Autodesk Fusion 360 part; units mm, degrees
note: some values were not read from the file. Set by a fixed rule: which sketch regions a step uses.
(part 3 of 3)
  spline S151 degree 3 poles (-49.2389, -12.8758) (-49.8818, -12.8354) (-50.64, -12.7486) (-51.5069, -12.5872) knots 0 0 0 0 1 1 1 1
  arc A152 (-51.6774, -11.868) -> (-51.5069, -12.5872) centre (0, 0) ccw
  spline S152 degree 3 poles (-51.6774, -11.868) (-50.9751, -11.3346) (-50.3365, -10.9168) (-49.7802, -10.5921) knots 0 0 0 0 1 1 1 1
  spline S153 degree 3 poles (-49.7802, -10.5921) (-49.639, -10.5097) (-49.5032, -10.4334) (-49.3731, -10.3628) knots 0 0 0 0 1 1 1 1
  arc A153 (-49.3731, -10.3628) -> (-49.172, -9.9321) centre (-49.564, -10.0113) ccw
  arc A154 (-49.276, -9.4025) -> (-49.172, -9.9321) centre (0, 0) ccw
  arc A155 (-49.276, -9.4025) -> (-49.6251, -9.0799) centre (-49.6689, -9.4775) ccw
  spline S154 degree 3 poles (-49.6251, -9.0799) (-49.7722, -9.0637) (-49.9268, -9.0443) (-50.0886, -9.0215) knots 0 0 0 0 1 1 1 1
  spline S155 degree 3 poles (-50.0886, -9.0215) (-50.7265, -8.9313) (-51.4757, -8.786) (-52.3275, -8.5579) knots 0 0 0 0 1 1 1 1
  arc A156 (-52.4417, -7.8277) -> (-52.3275, -8.5579) centre (0, 0) ccw
  spline S156 degree 3 poles (-52.4417, -7.8277) (-51.7002, -7.3504) (-51.0311, -6.9833) (-50.4513, -6.7027) knots 0 0 0 0 1 1 1 1
  spline S157 degree 3 poles (-50.4513, -6.7027) (-50.3042, -6.6315) (-50.1629, -6.5659) (-50.0277, -6.5056) knots 0 0 0 0 1 1 1 1
  arc A157 (-50.0277, -6.5056) -> (-49.7938, -6.0917) centre (-50.1908, -6.1403) ccw
  arc A158 (-49.8564, -5.5557) -> (-49.7938, -6.0917) centre (0, 0) ccw
  arc A159 (-49.8564, -5.5557) -> (-50.1795, -5.207) centre (-50.254, -5.6) ccw
  spline S158 degree 3 poles (-50.1795, -5.207) (-50.3249, -5.1794) (-50.4775, -5.1482) (-50.6371, -5.1128) knots 0 0 0 0 1 1 1 1
  spline S159 degree 3 poles (-50.6371, -5.1128) (-51.266, -4.9735) (-52.0017, -4.7706) (-52.8333, -4.4772) knots 0 0 0 0 1 1 1 1
  arc A160 (-52.8906, -3.7403) -> (-52.8333, -4.4772) centre (0, 0) ccw
  spline S160 degree 3 poles (-52.8906, -3.7403) (-52.1143, -3.3219) (-51.4188, -3.0078) (-50.819, -2.773) knots 0 0 0 0 1 1 1 1
  spline S161 degree 3 poles (-50.819, -2.773) (-50.6668, -2.7134) (-50.5208, -2.6589) (-50.3814, -2.6092) knots 0 0 0 0 1 1 1 1
  arc A161 (-50.3814, -2.6092) -> (-50.1161, -2.2148) centre (-50.5157, -2.2324) ccw
  arc A162 (-50.137, -1.6755) -> (-50.1161, -2.2148) centre (0, 0) ccw
  arc A163 (-50.137, -1.6755) -> (-50.4321, -1.3028) centre (-50.5368, -1.6888) ccw
  spline S162 degree 3 poles (-50.4321, -1.3028) (-50.5749, -1.2641) (-50.7247, -1.2211) (-50.881, -1.1735) knots 0 0 0 0 1 1 1 1
  spline S163 degree 3 poles (-50.881, -1.1735) (-51.4973, -0.9858) (-52.215, -0.7265) (-53.0214, -0.3696) knots 0 0 0 0 1 1 1 1
  arc A164 (-53.0214, 0.3696) -> (-53.0214, -0.3696) centre (0, 0) ccw
  spline S164 degree 3 poles (-53.0214, 0.3696) (-52.215, 0.7265) (-51.4973, 0.9858) (-50.881, 1.1735) knots 0 0 0 0 1 1 1 1
  spline S165 degree 3 poles (-50.881, 1.1735) (-50.7247, 1.2211) (-50.5749, 1.2641) (-50.4321, 1.3028) knots 0 0 0 0 1 1 1 1
  arc A165 (-50.4321, 1.3028) -> (-50.137, 1.6755) centre (-50.5368, 1.6888) ccw
  arc A166 (-50.1161, 2.2148) -> (-50.137, 1.6755) centre (0, 0) ccw
  arc A167 (-50.1161, 2.2148) -> (-50.3814, 2.6092) centre (-50.5157, 2.2324) ccw
  spline S166 degree 3 poles (-50.3814, 2.6092) (-50.5208, 2.6589) (-50.6668, 2.7134) (-50.819, 2.773) knots 0 0 0 0 1 1 1 1
  spline S167 degree 3 poles (-50.819, 2.773) (-51.4188, 3.0078) (-52.1143, 3.3219) (-52.8906, 3.7403) knots 0 0 0 0 1 1 1 1
  arc A168 (-52.8333, 4.4772) -> (-52.8906, 3.7403) centre (0, 0) ccw
  spline S168 degree 3 poles (-52.8333, 4.4772) (-52.0017, 4.7706) (-51.266, 4.9735) (-50.6371, 5.1128) knots 0 0 0 0 1 1 1 1
  spline S169 degree 3 poles (-50.6371, 5.1128) (-50.4775, 5.1482) (-50.3249, 5.1794) (-50.1795, 5.207) knots 0 0 0 0 1 1 1 1
  arc A169 (-50.1795, 5.207) -> (-49.8564, 5.5557) centre (-50.254, 5.6) ccw
  arc A170 (-49.7938, 6.0917) -> (-49.8564, 5.5557) centre (0, 0) ccw
  arc A171 (-49.7938, 6.0917) -> (-50.0277, 6.5056) centre (-50.1908, 6.1403) ccw
  spline S170 degree 3 poles (-50.0277, 6.5056) (-50.1629, 6.5659) (-50.3042, 6.6315) (-50.4513, 6.7027) knots 0 0 0 0 1 1 1 1
  spline S171 degree 3 poles (-50.4513, 6.7027) (-51.0311, 6.9833) (-51.7002, 7.3504) (-52.4417, 7.8277) knots 0 0 0 0 1 1 1 1
  arc A172 (-52.3275, 8.5579) -> (-52.4417, 7.8277) centre (0, 0) ccw
  spline S172 degree 3 poles (-52.3275, 8.5579) (-51.4757, 8.786) (-50.7265, 8.9313) (-50.0886, 9.0215) knots 0 0 0 0 1 1 1 1
  spline S173 degree 3 poles (-50.0886, 9.0215) (-49.9268, 9.0443) (-49.7722, 9.0637) (-49.6251, 9.0799) knots 0 0 0 0 1 1 1 1
  arc A173 (-49.6251, 9.0799) -> (-49.276, 9.4025) centre (-49.6689, 9.4775) ccw
  arc A174 (-49.172, 9.9321) -> (-49.276, 9.4025) centre (0, 0) ccw
  arc A175 (-49.172, 9.9321) -> (-49.3731, 10.3628) centre (-49.564, 10.0113) ccw
  spline S174 degree 3 poles (-49.3731, 10.3628) (-49.5032, 10.4334) (-49.639, 10.5097) (-49.7802, 10.5921) knots 0 0 0 0 1 1 1 1
  spline S175 degree 3 poles (-49.7802, 10.5921) (-50.3365, 10.9168) (-50.9751, 11.3346) (-51.6774, 11.868) knots 0 0 0 0 1 1 1 1
  arc A176 (-51.5069, 12.5872) -> (-51.6774, 11.868) centre (0, 0) ccw
  spline S176 degree 3 poles (-51.5069, 12.5872) (-50.64, 12.7486) (-49.8818, 12.8354) (-49.2389, 12.8758) knots 0 0 0 0 1 1 1 1
  spline S177 degree 3 poles (-49.2389, 12.8758) (-49.0758, 12.8861) (-48.9202, 12.8934) (-48.7722, 12.8981) knots 0 0 0 0 1 1 1 1
  arc A177 (-48.7722, 12.8981) -> (-48.3992, 13.1927) centre (-48.7851, 13.2979) ccw
  arc A178 (-48.2544, 13.7127) -> (-48.3992, 13.1927) centre (0, 0) ccw
  arc A179 (-48.2544, 13.7127) -> (-48.4216, 14.1576) centre (-48.6392, 13.822) ccw
  spline S178 degree 3 poles (-48.4216, 14.1576) (-48.5458, 14.2382) (-48.6753, 14.3248) (-48.8097, 14.4179) knots 0 0 0 0 1 1 1 1
  spline S179 degree 3 poles (-48.8097, 14.4179) (-49.3392, 14.7847) (-49.9435, 15.2507) (-50.6023, 15.8369) knots 0 0 0 0 1 1 1 1
  arc A180 (-50.3766, 16.5407) -> (-50.6023, 15.8369) centre (0, 0) ccw
  spline S180 degree 3 poles (-50.3766, 16.5407) (-49.4998, 16.6345) (-48.7372, 16.6622) (-48.0931, 16.6527) knots 0 0 0 0 1 1 1 1
  spline S181 degree 3 poles (-48.0931, 16.6527) (-47.9296, 16.6503) (-47.7739, 16.6455) (-47.6261, 16.6388) knots 0 0 0 0 1 1 1 1
  arc A181 (-47.6261, 16.6388) -> (-47.2313, 16.9036) centre (-47.6079, 17.0384) ccw
  arc A182 (-47.0467, 17.4108) -> (-47.2313, 16.9036) centre (0, 0) ccw
  arc A183 (-47.0467, 17.4108) -> (-47.1789, 17.8674) centre (-47.4218, 17.5496) ccw
  spline S182 degree 3 poles (-47.1789, 17.8674) (-47.2965, 17.9573) (-47.4189, 18.0537) (-47.5456, 18.1569) knots 0 0 0 0 1 1 1 1
  spline S183 degree 3 poles (-47.5456, 18.1569) (-48.0451, 18.5637) (-48.6115, 19.0751) (-49.2229, 19.7105) knots 0 0 0 0 1 1 1 1
  arc A184 (-48.9434, 20.3948) -> (-49.2229, 19.7105) centre (0, 0) ccw
  spline S184 degree 3 poles (-48.9434, 20.3948) (-48.0619, 20.4203) (-47.2994, 20.3889) (-46.658, 20.3295) knots 0 0 0 0 1 1 1 1
  spline S185 degree 3 poles (-46.658, 20.3295) (-46.4952, 20.3145) (-46.3404, 20.2976) (-46.1935, 20.2794) knots 0 0 0 0 1 1 1 1
  arc A185 (-46.1935, 20.2794) -> (-45.7794, 20.5129) centre (-46.1444, 20.6764) ccw
  arc A186 (-45.556, 21.0042) -> (-45.7794, 20.5129) centre (0, 0) ccw
  arc A187 (-45.556, 21.0042) -> (-45.6525, 21.4697) centre (-45.9193, 21.1717) ccw
  spline S186 degree 3 poles (-45.6525, 21.4697) (-45.7627, 21.5684) (-45.8773, 21.674) (-45.9956, 21.7867) knots 0 0 0 0 1 1 1 1
  spline S187 degree 3 poles (-45.9956, 21.7867) (-46.4621, 22.231) (-46.9871, 22.7848) (-47.5475, 23.4657) knots 0 0 0 0 1 1 1 1
  arc A188 (-47.2158, 24.1262) -> (-47.5475, 23.4657) centre (0, 0) ccw
  spline S188 degree 3 poles (-47.2158, 24.1262) (-46.335, 24.0833) (-45.5772, 23.9929) (-44.9423, 23.884) knots 0 0 0 0 1 1 1 1
  spline S189 degree 3 poles (-44.9423, 23.884) (-44.7812, 23.8564) (-44.6281, 23.8276) (-44.4831, 23.7981) knots 0 0 0 0 1 1 1 1
  arc A189 (-44.4831, 23.7981) -> (-44.0521, 23.9987) centre (-44.4034, 24.1901) ccw
  arc A190 (-43.7914, 24.4713) -> (-44.0521, 23.9987) centre (0, 0) ccw
  arc A191 (-43.7914, 24.4713) -> (-43.8514, 24.9428) centre (-44.1406, 24.6664) ccw
  spline S190 degree 3 poles (-43.8514, 24.9428) (-43.9537, 25.0498) (-44.0597, 25.164) (-44.169, 25.2855) knots 0 0 0 0 1 1 1 1
  spline S191 degree 3 poles (-44.169, 25.2855) (-44.5997, 25.7646) (-45.0802, 26.3574) (-45.5861, 27.0797) knots 0 0 0 0 1 1 1 1
  arc A192 (-45.2042, 27.7125) -> (-45.5861, 27.0797) centre (0, 0) ccw
  spline S192 degree 3 poles (-45.2042, 27.7125) (-44.3294, 27.6015) (-43.5809, 27.4527) (-42.9563, 27.2949) knots 0 0 0 0 1 1 1 1
  spline S193 degree 3 poles (-42.9563, 27.2949) (-42.7979, 27.2549) (-42.6475, 27.2143) (-42.5051, 27.1736) knots 0 0 0 0 1 1 1 1
  arc A193 (-42.5051, 27.1736) -> (-42.0599, 27.3403) centre (-42.3953, 27.5583) ccw
  arc A194 (-41.7634, 27.7912) -> (-42.0599, 27.3403) centre (0, 0) ccw
  arc A195 (-41.7634, 27.7912) -> (-41.7867, 28.266) centre (-42.0964, 28.0128) ccw
  spline S194 degree 3 poles (-41.7867, 28.266) (-41.8804, 28.3806) (-41.9772, 28.5026) (-42.0767, 28.6322) knots 0 0 0 0 1 1 1 1
  spline S195 degree 3 poles (-42.0767, 28.6322) (-42.469, 29.1432) (-42.9021, 29.7715) (-43.3505, 30.5308) knots 0 0 0 0 1 1 1 1
  arc A196 (-42.9207, 31.1322) -> (-43.3505, 30.5308) centre (0, 0) ccw
  spline S196 degree 3 poles (-42.9207, 31.1322) (-42.0572, 30.9537) (-41.3225, 30.7473) (-40.712, 30.5416) knots 0 0 0 0 1 1 1 1
  spline S197 degree 3 poles (-40.712, 30.5416) (-40.5571, 30.4894) (-40.4103, 30.4373) (-40.2716, 30.3858) knots 0 0 0 0 1 1 1 1
  arc A197 (-40.2716, 30.3858) -> (-39.8148, 30.5174) centre (-40.1323, 30.7607) ccw
  arc A198 (-39.4842, 30.944) -> (-39.8148, 30.5174) centre (0, 0) ccw
  arc A199 (-39.4842, 30.944) -> (-39.4706, 31.4191) centre (-39.799, 31.1907) ccw
  spline S198 degree 3 poles (-39.4706, 31.4191) (-39.5552, 31.5406) (-39.6423, 31.6698) (-39.7314, 31.8068) knots 0 0 0 0 1 1 1 1
  spline S199 degree 3 poles (-39.7314, 31.8068) (-40.0829, 32.3466) (-40.466, 33.0066) (-40.8543, 33.7984) knots 0 0 0 0 1 1 1 1
  arc A200 (-40.3792, 34.3646) -> (-40.8543, 33.7984) centre (0, 0) ccw
  spline S200 degree 3 poles (-40.3792, 34.3646) (-39.532, 34.1197) (-38.8155, 33.857) (-38.2228, 33.6046) knots 0 0 0 0 1 1 1 1
  spline S201 degree 3 poles (-38.2228, 33.6046) (-38.0725, 33.5406) (-37.9301, 33.4773) (-37.7958, 33.4151) knots 0 0 0 0 1 1 1 1
  arc A201 (-37.7958, 33.4151) -> (-37.3302, 33.511) centre (-37.6279, 33.7782) ccw
  arc A202 (-36.9675, 33.9106) -> (-37.3302, 33.511) centre (0, 0) ccw
  arc A203 (-36.9675, 33.9106) -> (-36.9172, 34.3833) centre (-37.2623, 34.181) ccw
  spline S202 degree 3 poles (-36.9172, 34.3833) (-36.9921, 34.511) (-37.0689, 34.6465) (-37.1472, 34.79) knots 0 0 0 0 1 1 1 1
  spline S203 degree 3 poles (-37.1472, 34.79) (-37.4558, 35.3555) (-37.7866, 36.0432) (-38.1123, 36.8626) knots 0 0 0 0 1 1 1 1
  arc A204 (-37.5947, 37.3903) -> (-38.1123, 36.8626) centre (0, 0) ccw
  spline S204 degree 3 poles (-37.5947, 37.3903) (-36.7691, 37.0806) (-36.0751, 36.7631) (-35.5038, 36.4656) knots 0 0 0 0 1 1 1 1
  spline S205 degree 3 poles (-35.5038, 36.4656) (-35.3588, 36.3901) (-35.2218, 36.3159) (-35.0927, 36.2435) knots 0 0 0 0 1 1 1 1
  arc A205 (-35.0927, 36.2435) -> (-34.6211, 36.303) centre (-34.8972, 36.5925) ccw
  arc A206 (-34.2285, 36.6734) -> (-34.6211, 36.303) centre (0, 0) ccw
  arc A207 (-34.2285, 36.6734) -> (-34.1418, 37.1407) centre (-34.5015, 36.9658) ccw
  spline S206 degree 3 poles (-34.1418, 37.1407) (-34.2065, 37.2738) (-34.2726, 37.4149) (-34.3395, 37.564) knots 0 0 0 0 1 1 1 1
  spline S207 degree 3 poles (-34.3395, 37.564) (-34.6033, 38.1517) (-34.8799, 38.863) (-35.1411, 39.7052) knots 0 0 0 0 1 1 1 1
  arc A208 (-34.5842, 40.1912) -> (-35.1411, 39.7052) centre (0, 0) ccw
  spline S208 degree 3 poles (-34.5842, 40.1912) (-33.7851, 39.8184) (-33.1178, 39.4481) (-32.5712, 39.1072) knots 0 0 0 0 1 1 1 1
  spline S209 degree 3 poles (-32.5712, 39.1072) (-32.4326, 39.0207) (-32.3017, 38.9361) (-32.1786, 38.854) knots 0 0 0 0 1 1 1 1
  arc A209 (-32.1786, 38.854) -> (-31.7038, 38.8767) centre (-31.9566, 39.1867) ccw
  arc A210 (-31.2837, 39.2155) -> (-31.7038, 38.8767) centre (0, 0) ccw
  arc A211 (-31.2837, 39.2155) -> (-31.161, 39.6748) centre (-31.5331, 39.5282) ccw
  spline S210 degree 3 poles (-31.161, 39.6748) (-31.2152, 39.8125) (-31.2701, 39.9583) (-31.3253, 40.1121) knots 0 0 0 0 1 1 1 1
  spline S211 degree 3 poles (-31.3253, 40.1121) (-31.5428, 40.7185) (-31.7634, 41.449) (-31.9586, 42.309) knots 0 0 0 0 1 1 1 1
  arc A212 (-31.3657, 42.7504) -> (-31.9586, 42.309) centre (0, 0) ccw
  spline S212 degree 3 poles (-31.3657, 42.7504) (-30.5979, 42.3168) (-29.9613, 41.8959) (-29.4428, 41.5136) knots 0 0 0 0 1 1 1 1
  spline S213 degree 3 poles (-29.4428, 41.5136) (-29.3112, 41.4166) (-29.1873, 41.3222) (-29.071, 41.2307) knots 0 0 0 0 1 1 1 1
  arc A213 (-29.071, 41.2307) -> (-28.5958, 41.2166) centre (-28.8238, 41.5452) ccw
  arc A214 (-28.1507, 41.5219) -> (-28.5958, 41.2166) centre (0, 0) ccw
  arc A215 (-28.1507, 41.5219) -> (-27.9928, 41.9702) centre (-28.3752, 41.8529) ccw
  spline S214 degree 3 poles (-27.9928, 41.9702) (-28.0362, 42.1117) (-28.0796, 42.2613) (-28.1227, 42.419) knots 0 0 0 0 1 1 1 1
  spline S215 degree 3 poles (-28.1227, 42.419) (-28.2926, 43.0404) (-28.4559, 43.7858) (-28.5839, 44.6583) knots 0 0 0 0 1 1 1 1
  arc A216 (-27.9586, 45.0524) -> (-28.5839, 44.6583) centre (0, 0) ccw
  spline S216 degree 3 poles (-27.9586, 45.0524) (-27.2266, 44.5606) (-26.6246, 44.0917) (-26.1373, 43.6704) knots 0 0 0 0 1 1 1 1
  spline S217 degree 3 poles (-26.1373, 43.6704) (-26.0136, 43.5635) (-25.8974, 43.4597) (-25.7885, 43.3595) knots 0 0 0 0 1 1 1 1
  arc A217 (-25.7885, 43.3595) -> (-25.3158, 43.3086) centre (-25.5177, 43.6539) ccw
  arc A218 (-24.8484, 43.5785) -> (-25.3158, 43.3086) centre (0, 0) ccw
  arc A219 (-24.8484, 43.5785) -> (-24.6562, 44.0132) centre (-25.0466, 43.9259) ccw
  spline S218 degree 3 poles (-24.6562, 44.0132) (-24.6885, 44.1577) (-24.7203, 44.3102) (-24.751, 44.4707) knots 0 0 0 0 1 1 1 1
  spline S219 degree 3 poles (-24.751, 44.4707) (-24.8722, 45.1034) (-24.9773, 45.8593) (-25.0372, 46.739) knots 0 0 0 0 1 1 1 1
  arc A220 (-24.3833, 47.0835) -> (-25.0372, 46.739) centre (0, 0) ccw
  spline S220 degree 3 poles (-24.3833, 47.0835) (-23.6917, 46.5365) (-23.1277, 46.0223) (-22.6745, 45.5645) knots 0 0 0 0 1 1 1 1
  spline S221 degree 3 poles (-22.6745, 45.5645) (-22.5595, 45.4483) (-22.4517, 45.3359) (-22.3509, 45.2276) knots 0 0 0 0 1 1 1 1
  arc A221 (-22.3509, 45.2276) -> (-21.8836, 45.1402) centre (-22.0581, 45.5001) ccw
  arc A222 (-21.3967, 45.373) -> (-21.8836, 45.1402) centre (0, 0) ccw
  arc A223 (-21.3967, 45.373) -> (-21.1714, 45.7916) centre (-21.5673, 45.7348) ccw
  spline S222 degree 3 poles (-21.1714, 45.7916) (-21.1924, 45.9381) (-21.2122, 46.0926) (-21.2304, 46.255) knots 0 0 0 0 1 1 1 1
  spline S223 degree 3 poles (-21.2304, 46.255) (-21.3023, 46.8952) (-21.3484, 47.6569) (-21.34, 48.5387) knots 0 0 0 0 1 1 1 1
  arc A224 (-20.6613, 48.8314) -> (-21.34, 48.5387) centre (0, 0) ccw
  spline S224 degree 3 poles (-20.6613, 48.8314) (-20.0142, 48.2325) (-19.4918, 47.6761) (-19.0754, 47.1846) knots 0 0 0 0 1 1 1 1
  spline S225 degree 3 poles (-19.0754, 47.1846) (-18.9698, 47.0599) (-18.871, 46.9394) (-18.7789, 46.8236) knots 0 0 0 0 1 1 1 1
  arc A225 (-18.7789, 46.8236) -> (-18.3198, 46.7002) centre (-18.4659, 47.0726) ccw
  arc A226 (-17.8163, 46.8946) -> (-18.3198, 46.7002) centre (0, 0) ccw
  arc A227 (-17.8163, 46.8946) -> (-17.5592, 47.2945) centre (-17.9584, 47.2686) ccw
  spline S226 degree 3 poles (-17.5592, 47.2945) (-17.5688, 47.4422) (-17.5766, 47.5978) (-17.5822, 47.7611) knots 0 0 0 0 1 1 1 1
  spline S227 degree 3 poles (-17.5822, 47.7611) (-17.6042, 48.4049) (-17.5912, 49.1679) (-17.5145, 50.0464) knots 0 0 0 0 1 1 1 1
  arc A228 (-16.8151, 50.2857) -> (-17.5145, 50.0464) centre (0, 0) ccw
  spline S228 degree 3 poles (-16.8151, 50.2857) (-16.2164, 49.6384) (-15.7387, 49.0432) (-15.3616, 48.5209) knots 0 0 0 0 1 1 1 1
  spline S229 degree 3 poles (-15.3616, 48.5209) (-15.266, 48.3884) (-15.1768, 48.2606) (-15.0939, 48.138) knots 0 0 0 0 1 1 1 1
  arc A229 (-15.0939, 48.138) -> (-14.6458, 47.9795) centre (-14.7626, 48.362) ccw
  arc A230 (-14.1288, 48.1342) -> (-14.6458, 47.9795) centre (0, 0) ccw
  arc A231 (-14.1288, 48.1342) -> (-13.8415, 48.513) centre (-14.2414, 48.5181) ccw
  spline S230 degree 3 poles (-13.8415, 48.513) (-13.8396, 48.661) (-13.8353, 48.8167) (-13.8282, 48.98) knots 0 0 0 0 1 1 1 1
  spline S231 degree 3 poles (-13.8282, 48.98) (-13.8002, 49.6236) (-13.7282, 50.3833) (-13.5836, 51.2532) knots 0 0 0 0 1 1 1 1
  arc A232 (-12.8678, 51.4375) -> (-13.5836, 51.2532) centre (0, 0) ccw
  spline S232 degree 3 poles (-12.8678, 51.4375) (-12.321, 50.7457) (-11.8909, 50.1154) (-11.5554, 49.5654) knots 0 0 0 0 1 1 1 1
  spline S233 degree 3 poles (-11.5554, 49.5654) (-11.4703, 49.4259) (-11.3914, 49.2916) (-11.3182, 49.1629) knots 0 0 0 0 1 1 1 1
  arc A233 (-11.3182, 49.1629) -> (-10.8837, 48.9701) centre (-10.9705, 49.3606) ccw
  arc A234 (-10.3562, 49.0844) -> (-10.8837, 48.9701) centre (0, 0) ccw
  arc A235 (-10.3562, 49.0844) -> (-10.0404, 49.4397) centre (-10.4388, 49.4758) ccw
  spline S234 degree 3 poles (-10.0404, 49.4397) (-10.0271, 49.5871) (-10.0108, 49.742) (-9.991, 49.9043) knots 0 0 0 0 1 1 1 1
  spline S235 degree 3 poles (-9.991, 49.9043) (-9.9133, 50.5437) (-9.7826, 51.2956) (-9.571, 52.1517) knots 0 0 0 0 1 1 1 1
  arc A236 (-8.8431, 52.28) -> (-9.571, 52.1517) centre (0, 0) ccw
  spline S236 degree 3 poles (-8.8431, 52.28) (-8.3515, 51.5479) (-7.9715, 50.8861) (-7.6798, 50.3118) knots 0 0 0 0 1 1 1 1
  spline S237 degree 3 poles (-7.6798, 50.3118) (-7.6057, 50.1661) (-7.5374, 50.0261) (-7.4744, 49.8921) knots 0 0 0 0 1 1 1 1
  arc A237 (-7.4744, 49.8921) -> (-7.0562, 49.6663) centre (-7.1124, 50.0623) ccw
  arc A238 (-6.5214, 49.7393) -> (-7.0562, 49.6663) centre (0, 0) ccw
  arc A239 (-6.5214, 49.7393) -> (-6.1791, 50.0691) centre (-6.5734, 50.1359) ccw
  spline S238 degree 3 poles (-6.1791, 50.0691) (-6.1543, 50.215) (-6.1261, 50.3682) (-6.0938, 50.5284) knots 0 0 0 0 1 1 1 1
  spline S239 degree 3 poles (-6.0938, 50.5284) (-5.9667, 51.16) (-5.7781, 51.8994) (-5.5009, 52.7365) knots 0 0 0 0 1 1 1 1
  arc A240 (-4.7652, 52.8081) -> (-5.5009, 52.7365) centre (0, 0) ccw
  spline S240 degree 3 poles (-4.7652, 52.8081) (-4.3318, 52.0401) (-4.0043, 51.3508) (-3.7579, 50.7556) knots 0 0 0 0 1 1 1 1
  spline S241 degree 3 poles (-3.7579, 50.7556) (-3.6953, 50.6046) (-3.6381, 50.4598) (-3.5857, 50.3213) knots 0 0 0 0 1 1 1 1
  arc A241 (-3.5857, 50.3213) -> (-3.1862, 50.0637) centre (-3.2116, 50.4629) ccw
  arc A242 (-2.6474, 50.0951) -> (-3.1862, 50.0637) centre (0, 0) ccw
  arc A243 (-2.6474, 50.0951) -> (-2.2805, 50.3974) centre (-2.6685, 50.4945) ccw
  spline S242 degree 3 poles (-2.2805, 50.3974) (-2.2445, 50.5409) (-2.2045, 50.6915) (-2.1599, 50.8487) knots 0 0 0 0 1 1 1 1
  spline S243 degree 3 poles (-2.1599, 50.8487) (-1.9843, 51.4685) (-1.7389, 52.1911) (-1.3977, 53.0042) knots 0 0 0 0 1 1 1 1
  arc A244 (-0.6587, 53.0186) -> (-1.3977, 53.0042) centre (0, 0) ccw
  spline S244 degree 3 poles (-0.6587, 53.0186) (-0.2861, 52.2193) (-0.0129, 51.5067) (0.1866, 50.8942) knots 0 0 0 0 1 1 1 1
  spline S245 degree 3 poles (0.1866, 50.8942) (0.2372, 50.7388) (0.2831, 50.59) (0.3246, 50.4479) knots 0 0 0 0 1 1 1 1
  arc A245 (0.3246, 50.4479) -> (0.703, 50.1601) centre (0.7086, 50.56) ccw
  arc A246 (1.2426, 50.1496) -> (0.703, 50.1601) centre (0, 0) ccw
  arc A247 (1.2426, 50.1496) -> (1.6318, 50.4225) centre (1.2525, 50.5495) ccw
  spline S246 degree 3 poles (1.6318, 50.4225) (1.6788, 50.5629) (1.7304, 50.7099) (1.787, 50.8632) knots 0 0 0 0 1 1 1 1
  spline S247 degree 3 poles (1.787, 50.8632) (2.0101, 51.4675) (2.3107, 52.1689) (2.714, 52.9531) knots 0 0 0 0 1 1 1 1
  arc A248 (3.4519, 52.9102) -> (2.714, 52.9531) centre (0, 0) ccw
  spline S248 degree 3 poles (3.4519, 52.9102) (3.7614, 52.0844) (3.9785, 51.3529) (4.13, 50.7267) knots 0 0 0 0 1 1 1 1
  spline S249 degree 3 poles (4.13, 50.7267) (4.1684, 50.5679) (4.2026, 50.4159) (4.233, 50.271) knots 0 0 0 0 1 1 1 1
  arc A249 (4.233, 50.271) -> (4.5879, 49.9548) centre (4.6244, 50.3531) ccw
  arc A250 (5.125, 49.9025) -> (4.5879, 49.9548) centre (0, 0) ccw
  arc A251 (5.125, 49.9025) -> (5.5342, 50.1445) centre (5.1659, 50.3004) ccw
  spline S250 degree 3 poles (5.5342, 50.1445) (5.5919, 50.2807) (5.6548, 50.4233) (5.7231, 50.5718) knots 0 0 0 0 1 1 1 1
  spline S251 degree 3 poles (5.7231, 50.5718) (5.9924, 51.157) (6.3465, 51.833) (6.8093, 52.5836) knots 0 0 0 0 1 1 1 1
  arc A252 (7.5416, 52.4836) -> (6.8093, 52.5836) centre (0, 0) ccw
  spline S252 degree 3 poles (7.5416, 52.4836) (7.7862, 51.6363) (7.946, 50.8901) (8.0485, 50.2541) knots 0 0 0 0 1 1 1 1
  spline S253 degree 3 poles (8.0485, 50.2541) (8.0745, 50.0928) (8.0968, 49.9386) (8.1159, 49.7918) knots 0 0 0 0 1 1 1 1
  arc A253 (8.1159, 49.7918) -> (8.4452, 49.449) centre (8.5125, 49.8433) ccw
  arc A254 (8.9767, 49.3553) -> (8.4452, 49.449) centre (0, 0) ccw
  arc A255 (8.9767, 49.3553) -> (9.4034, 49.5648) centre (9.0483, 49.7489) ccw
  spline S254 degree 3 poles (9.4034, 49.5648) (9.4715, 49.6962) (9.5452, 49.8335) (9.6248, 49.9762) knots 0 0 0 0 1 1 1 1
  spline S255 degree 3 poles (9.6248, 49.9762) (9.9387, 50.5388) (10.344, 51.1853) (10.8636, 51.8978) knots 0 0 0 0 1 1 1 1
  arc A256 (11.586, 51.7413) -> (10.8636, 51.8978) centre (0, 0) ccw
  spline S256 degree 3 poles (11.586, 51.7413) (11.7642, 50.8777) (11.8657, 50.1213) (11.9186, 49.4793) knots 0 0 0 0 1 1 1 1
  spline S257 degree 3 poles (11.9186, 49.4793) (11.932, 49.3164) (11.9423, 49.161) (11.9499, 49.0132) knots 0 0 0 0 1 1 1 1
  arc A257 (11.9499, 49.0132) -> (12.2517, 48.6459) centre (12.3494, 49.0338) ccw
  arc A258 (12.7744, 48.5113) -> (12.2517, 48.6459) centre (0, 0) ccw
  arc A259 (12.7744, 48.5113) -> (13.216, 48.6871) centre (12.8762, 48.8981) ccw
  spline S258 degree 3 poles (13.216, 48.6871) (13.2941, 48.8128) (13.3782, 48.9439) (13.4687, 49.0801) knots 0 0 0 0 1 1 1 1
  spline S259 degree 3 poles (13.4687, 49.0801) (13.8252, 49.6166) (14.2794, 50.2298) (14.8527, 50.8999) knots 0 0 0 0 1 1 1 1
  arc A260 (15.5607, 50.6879) -> (14.8527, 50.8999) centre (0, 0) ccw
  spline S260 degree 3 poles (15.5607, 50.6879) (15.6715, 49.8131) (15.714, 49.0511) (15.717, 48.4069) knots 0 0 0 0 1 1 1 1
  spline S261 degree 3 poles (15.717, 48.4069) (15.7178, 48.2435) (15.716, 48.0877) (15.7122, 47.9398) knots 0 0 0 0 1 1 1 1
  arc A261 (15.7122, 47.9398) -> (15.9846, 47.5502) centre (16.112, 47.9294) ccw
  arc A262 (16.4952, 47.3755) -> (15.9846, 47.5502) centre (0, 0) ccw
  arc A263 (16.4952, 47.3755) -> (16.9492, 47.5165) centre (16.6267, 47.7532) ccw
  spline S262 degree 3 poles (16.9492, 47.5165) (17.0368, 47.6358) (17.1308, 47.76) (17.2315, 47.8887) knots 0 0 0 0 1 1 1 1
  spline S263 degree 3 poles (17.2315, 47.8887) (17.6285, 48.3961) (18.1289, 48.9722) (18.7523, 49.5959) knots 0 0 0 0 1 1 1 1
  arc A264 (19.4419, 49.3297) -> (18.7523, 49.5959) centre (0, 0) ccw
  spline S264 degree 3 poles (19.4419, 49.3297) (19.4845, 48.4489) (19.4679, 47.6859) (19.4209, 47.0434) knots 0 0 0 0 1 1 1 1
  spline S265 degree 3 poles (19.4209, 47.0434) (19.409, 46.8804) (19.3952, 46.7253) (19.3799, 46.578) knots 0 0 0 0 1 1 1 1
  arc A265 (19.3799, 46.578) -> (19.6213, 46.1685) centre (19.7777, 46.5367) ccw
  arc A266 (20.1168, 45.9548) -> (19.6213, 46.1685) centre (0, 0) ccw
  arc A267 (20.1168, 45.9548) -> (20.5804, 46.0602) centre (20.2772, 46.3212) ccw
  spline S266 degree 3 poles (20.5804, 46.0602) (20.6769, 46.1724) (20.7803, 46.2889) (20.8907, 46.4094) knots 0 0 0 0 1 1 1 1
  spline S267 degree 3 poles (20.8907, 46.4094) (21.3258, 46.8845) (21.8694, 47.4201) (22.5393, 47.9936) knots 0 0 0 0 1 1 1 1
  arc A268 (23.2061, 47.6747) -> (22.5393, 47.9936) centre (0, 0) ccw
  spline S268 degree 3 poles (23.2061, 47.6747) (23.1803, 46.7933) (23.1046, 46.0339) (23.008, 45.397) knots 0 0 0 0 1 1 1 1
  spline S269 degree 3 poles (23.008, 45.397) (22.9835, 45.2354) (22.9577, 45.0818) (22.931, 44.9362) knots 0 0 0 0 1 1 1 1
  arc A269 (22.931, 44.9362) -> (23.14, 44.5092) centre (23.3245, 44.8641) ccw
  arc A270 (23.6175, 44.2577) -> (23.14, 44.5092) centre (0, 0) ccw
  arc A271 (23.6175, 44.2577) -> (24.0878, 44.3269) centre (23.8058, 44.6106) ccw
  spline S270 degree 3 poles (24.0878, 44.3269) (24.1928, 44.4312) (24.3048, 44.5394) (24.4243, 44.651) knots 0 0 0 0 1 1 1 1
  spline S271 degree 3 poles (24.4243, 44.651) (24.8949, 45.0909) (25.4783, 45.5828) (26.1906, 46.1026) knots 0 0 0 0 1 1 1 1
  arc A272 (26.8307, 45.7331) -> (26.1906, 46.1026) centre (0, 0) ccw
  spline S272 degree 3 poles (26.8307, 45.7331) (26.7367, 44.8563) (26.6024, 44.105) (26.4568, 43.4775) knots 0 0 0 0 1 1 1 1
  spline S273 degree 3 poles (26.4568, 43.4775) (26.4198, 43.3183) (26.3822, 43.1672) (26.3443, 43.0241) knots 0 0 0 0 1 1 1 1
  arc A273 (26.3443, 43.0241) -> (26.5195, 42.5822) centre (26.731, 42.9217) ccw
  arc A274 (26.9761, 42.2944) -> (26.5195, 42.5822) centre (0, 0) ccw
  arc A275 (26.9761, 42.2944) -> (27.4504, 42.327) centre (27.1912, 42.6317) ccw
  spline S274 degree 3 poles (27.4504, 42.327) (27.5631, 42.4229) (27.6832, 42.522) (27.8109, 42.624) knots 0 0 0 0 1 1 1 1
  spline S275 degree 3 poles (27.8109, 42.624) (28.3142, 43.0261) (28.934, 43.4714) (29.6845, 43.9344) knots 0 0 0 0 1 1 1 1
  arc A276 (30.294, 43.5164) -> (29.6845, 43.9344) centre (0, 0) ccw
  spline S276 degree 3 poles (30.294, 43.5164) (30.1323, 42.6495) (29.9402, 41.9109) (29.7464, 41.2966) knots 0 0 0 0 1 1 1 1
  spline S277 degree 3 poles (29.7464, 41.2966) (29.6972, 41.1407) (29.648, 40.9929) (29.5991, 40.8532) knots 0 0 0 0 1 1 1 1
  arc A277 (29.5991, 40.8532) -> (29.7396, 40.3991) centre (29.9767, 40.7212) ccw
  arc A278 (30.1725, 40.0768) -> (29.7396, 40.3991) centre (0, 0) ccw
  arc A279 (30.1725, 40.0768) -> (30.6478, 40.0725) centre (30.4131, 40.3963) ccw
  spline S278 degree 3 poles (30.6478, 40.0725) (30.7677, 40.1594) (30.8951, 40.2489) (31.0303, 40.3407) knots 0 0 0 0 1 1 1 1
  spline S279 degree 3 poles (31.0303, 40.3407) (31.5633, 40.7026) (32.2157, 41.0985) (32.9998, 41.502) knots 0 0 0 0 1 1 1 1
  arc A280 (33.5751, 41.0379) -> (32.9998, 41.502) centre (0, 0) ccw
  spline S280 degree 3 poles (33.5751, 41.0379) (33.3467, 40.1862) (33.098, 39.4648) (32.8571, 38.8673) knots 0 0 0 0 1 1 1 1
  spline S281 degree 3 poles (32.8571, 38.8673) (32.796, 38.7157) (32.7355, 38.5722) (32.6759, 38.4367) knots 0 0 0 0 1 1 1 1
  arc A281 (32.6759, 38.4367) -> (32.7808, 37.973) centre (33.0422, 38.2758) ccw
  arc A282 (33.1874, 37.6181) -> (32.7808, 37.973) centre (0, 0) ccw
  arc A283 (33.1874, 37.6181) -> (33.661, 37.577) centre (33.452, 37.9181) ccw
  spline S282 degree 3 poles (33.661, 37.577) (33.7872, 37.6543) (33.9212, 37.7338) (34.0631, 37.8148) knots 0 0 0 0 1 1 1 1
  spline S283 degree 3 poles (34.0631, 37.8148) (34.6225, 38.1343) (35.3037, 38.4784) (36.1166, 38.82) knots 0 0 0 0 1 1 1 1
  arc A284 (36.6543, 38.3127) -> (36.1166, 38.82) centre (0, 0) ccw
  spline S284 degree 3 poles (36.6543, 38.3127) (36.3606, 37.4812) (36.0567, 36.7813) (35.7702, 36.2042) knots 0 0 0 0 1 1 1 1
  spline S285 degree 3 poles (35.7702, 36.2042) (35.6976, 36.0578) (35.6261, 35.9194) (35.5562, 35.7889) knots 0 0 0 0 1 1 1 1
  arc A285 (35.5562, 35.7889) -> (35.6248, 35.3186) centre (35.9089, 35.6002) ccw
  arc A286 (36.0027, 34.9332) -> (35.6248, 35.3186) centre (0, 0) ccw
  arc A287 (36.0027, 34.9332) -> (36.4717, 34.8555) centre (36.2898, 35.2118) ccw
  spline S286 degree 3 poles (36.4717, 34.8555) (36.6035, 34.9229) (36.7433, 34.9917) (36.8911, 35.0615) knots 0 0 0 0 1 1 1 1
  spline S287 degree 3 poles (36.8911, 35.0615) (37.4735, 35.3366) (38.1793, 35.627) (39.0163, 35.9045) knots 0 0 0 0 1 1 1 1
  arc A288 (39.513, 35.3571) -> (39.0163, 35.9045) centre (0, 0) ccw
  spline S288 degree 3 poles (39.513, 35.3571) (39.1558, 34.5509) (38.7985, 33.8765) (38.4682, 33.3234) knots 0 0 0 0 1 1 1 1
  spline S289 degree 3 poles (38.4682, 33.3234) (38.3844, 33.1831) (38.3024, 33.0507) (38.2227, 32.926) knots 0 0 0 0 1 1 1 1
  arc A289 (38.2227, 32.926) -> (38.2546, 32.4517) centre (38.5596, 32.7105) ccw
  arc A290 (38.6015, 32.0383) -> (38.2546, 32.4517) centre (0, 0) ccw
  arc A291 (38.6015, 32.0383) -> (39.0631, 31.9244) centre (38.9093, 32.2937) ccw
  spline S290 degree 3 poles (39.0631, 31.9244) (39.1997, 31.9813) (39.3444, 32.0391) (39.4971, 32.0973) knots 0 0 0 0 1 1 1 1
  spline S291 degree 3 poles (39.4971, 32.0973) (40.0992, 32.3265) (40.8253, 32.5612) (41.6813, 32.773) knots 0 0 0 0 1 1 1 1
  arc A292 (42.1341, 32.1888) -> (41.6813, 32.773) centre (0, 0) ccw
  spline S292 degree 3 poles (42.1341, 32.1888) (41.7155, 31.4127) (41.307, 30.7681) (40.9349, 30.2422) knots 0 0 0 0 1 1 1 1
  spline S293 degree 3 poles (40.9349, 30.2422) (40.8405, 30.1088) (40.7484, 29.9831) (40.6593, 29.865) knots 0 0 0 0 1 1 1 1
  arc A293 (40.6593, 29.865) -> (40.6543, 29.3897) centre (40.9785, 29.624) ccw
  arc A294 (40.9682, 28.9506) -> (40.6543, 29.3897) centre (0, 0) ccw
  arc A295 (40.9682, 28.9506) -> (41.4195, 28.8014) centre (41.2948, 29.1814) ccw
  spline S294 degree 3 poles (41.4195, 28.8014) (41.5601, 28.8475) (41.7089, 28.8939) (41.8657, 28.94) knots 0 0 0 0 1 1 1 1
  spline S295 degree 3 poles (41.8657, 28.94) (42.4836, 29.1219) (43.2258, 29.2997) (44.0956, 29.4445) knots 0 0 0 0 1 1 1 1
  arc A296 (44.5018, 28.8269) -> (44.0956, 29.4445) centre (0, 0) ccw
  spline S296 degree 3 poles (44.5018, 28.8269) (44.0243, 28.0856) (43.5671, 27.4746) (43.1553, 26.9792) knots 0 0 0 0 1 1 1 1
  spline S297 degree 3 poles (43.1553, 26.9792) (43.0509, 26.8535) (42.9494, 26.7353) (42.8513, 26.6244) knots 0 0 0 0 1 1 1 1
  arc A297 (42.8513, 26.6244) -> (42.8096, 26.1509) centre (43.1509, 26.3594) ccw
  arc A298 (43.0884, 25.6888) -> (42.8096, 26.1509) centre (0, 0) ccw
  arc A299 (43.0884, 25.6888) -> (43.5268, 25.5051) centre (43.432, 25.8936) ccw
  spline S298 degree 3 poles (43.5268, 25.5051) (43.6706, 25.5401) (43.8225, 25.5749) (43.9824, 25.6087) knots 0 0 0 0 1 1 1 1
  spline S299 degree 3 poles (43.9824, 25.6087) (44.6126, 25.7422) (45.3663, 25.8619) (46.2447, 25.9389) knots 0 0 0 0 1 1 1 1
  arc A300 (46.6018, 25.2917) -> (46.2447, 25.9389) centre (0, 0) ccw
  spline S300 degree 3 poles (46.6018, 25.2917) (46.0683, 24.5896) (45.5652, 24.0158) (45.1162, 23.5538) knots 0 0 0 0 1 1 1 1
  spline S301 degree 3 poles (45.1162, 23.5538) (45.0023, 23.4366) (44.892, 23.3266) (44.7856, 23.2237) knots 0 0 0 0 1 1 1 1
  arc A301 (44.7856, 23.2237) -> (44.7073, 22.7548) centre (45.0638, 22.9363) ccw
  arc A302 (44.9495, 22.2725) -> (44.7073, 22.7548) centre (0, 0) ccw
  arc A303 (44.9495, 22.2725) -> (45.3724, 22.0554) centre (45.308, 22.4501) ccw
  spline S302 degree 3 poles (45.3724, 22.0554) (45.5185, 22.0792) (45.6726, 22.102) (45.8346, 22.1234) knots 0 0 0 0 1 1 1 1
  spline S303 degree 3 poles (45.8346, 22.1234) (46.4733, 22.2076) (47.234, 22.2686) (48.1157, 22.2773) knots 0 0 0 0 1 1 1 1
  arc A304 (48.4216, 21.6044) -> (48.1157, 22.2773) centre (0, 0) ccw
  spline S304 degree 3 poles (48.4216, 21.6044) (47.8353, 20.9457) (47.2892, 20.4127) (46.8058, 19.9868) knots 0 0 0 0 1 1 1 1
  spline S305 degree 3 poles (46.8058, 19.9868) (46.6832, 19.8788) (46.5646, 19.7777) (46.4506, 19.6833) knots 0 0 0 0 1 1 1 1
  arc A305 (46.4506, 19.6833) -> (46.3362, 19.2219) centre (46.7057, 19.3752) ccw
  arc A306 (46.5403, 18.7223) -> (46.3362, 19.2219) centre (0, 0) ccw
  arc A307 (46.5403, 18.7223) -> (46.9451, 18.473) centre (46.9114, 18.8716) ccw
  spline S306 degree 3 poles (46.9451, 18.473) (47.0926, 18.4855) (47.248, 18.4963) (47.4112, 18.505) knots 0 0 0 0 1 1 1 1
  spline S307 degree 3 poles (47.4112, 18.505) (48.0545, 18.5395) (48.8176, 18.5413) (49.6974, 18.4817) knots 0 0 0 0 1 1 1 1
  arc A308 (49.9502, 17.7871) -> (49.6974, 18.4817) centre (0, 0) ccw
  spline S308 degree 3 poles (49.9502, 17.7871) (49.3146, 17.1759) (48.7288, 16.6867) (48.2139, 16.2996) knots 0 0 0 0 1 1 1 1
  spline S309 degree 3 poles (48.2139, 16.2996) (48.0832, 16.2014) (47.9572, 16.1098) (47.8363, 16.0246) knots 0 0 0 0 1 1 1 1
  arc A309 (47.8363, 16.0246) -> (47.6864, 15.5734) centre (48.0667, 15.6976) ccw
  arc A310 (47.8512, 15.0595) -> (47.6864, 15.5734) centre (0, 0) ccw
  arc A311 (47.8512, 15.0595) -> (48.2354, 14.7796) centre (48.2328, 15.1796) ccw
  spline S310 degree 3 poles (48.2354, 14.7796) (48.3834, 14.7806) (48.5392, 14.7793) (48.7026, 14.7754) knots 0 0 0 0 1 1 1 1
  spline S311 degree 3 poles (48.7026, 14.7754) (49.3466, 14.7599) (50.1076, 14.7026) (50.9801, 14.5749) knots 0 0 0 0 1 1 1 1
  arc A312 (51.1783, 13.8628) -> (50.9801, 14.5749) centre (0, 0) ccw
  spline S312 degree 3 poles (51.1783, 13.8628) (50.4973, 13.3027) (49.8754, 12.8604) (49.332, 12.5144) knots 0 0 0 0 1 1 1 1
  spline S313 degree 3 poles (49.332, 12.5144) (49.1941, 12.4266) (49.0614, 12.3451) (48.9342, 12.2694) knots 0 0 0 0 1 1 1 1
  arc A313 (48.9342, 12.2694) -> (48.7499, 11.8313) centre (49.1386, 11.9256) ccw
  arc A314 (48.8743, 11.3061) -> (48.7499, 11.8313) centre (0, 0) ccw
  arc A315 (48.8743, 11.3061) -> (49.2357, 10.9973) centre (49.264, 11.3963) ccw
  spline S314 degree 3 poles (49.2357, 10.9973) (49.3833, 10.9868) (49.5385, 10.9735) (49.7011, 10.9569) knots 0 0 0 0 1 1 1 1
  spline S315 degree 3 poles (49.7011, 10.9569) (50.342, 10.8915) (51.0963, 10.7754) (51.9563, 10.5805) knots 0 0 0 0 1 1 1 1
  arc A316 (52.0987, 9.8552) -> (51.9563, 10.5805) centre (0, 0) ccw
  spline S316 degree 3 poles (52.0987, 9.8552) (51.3763, 9.3495) (50.722, 8.9568) (50.1534, 8.6539) knots 0 0 0 0 1 1 1 1
  spline S317 degree 3 poles (50.1534, 8.6539) (50.0092, 8.5771) (49.8705, 8.5061) (49.7378, 8.4405) knots 0 0 0 0 1 1 1 1
  arc A317 (49.7378, 8.4405) -> (49.5201, 8.0179) centre (49.915, 8.0819) ccw
  arc A318 (49.6035, 7.4847) -> (49.5201, 8.0179) centre (0, 0) ccw
  arc A319 (49.6035, 7.4847) -> (49.9398, 7.1488) centre (49.999, 7.5444) ccw
  spline S318 degree 3 poles (49.9398, 7.1488) (50.0862, 7.1269) (50.2399, 7.1016) (50.4008, 7.0725) knots 0 0 0 0 1 1 1 1
  spline S319 degree 3 poles (50.4008, 7.0725) (51.0346, 6.9576) (51.7776, 6.7834) (52.6199, 6.5225) knots 0 0 0 0 1 1 1 1
  arc A320 (52.7058, 5.7883) -> (52.6199, 6.5225) centre (0, 0) ccw
  spline S320 degree 3 poles (52.7058, 5.7883) (51.9463, 5.3402) (51.2635, 4.9993) (50.6732, 4.7414) knots 0 0 0 0 1 1 1 1
  spline S321 degree 3 poles (50.6732, 4.7414) (50.5235, 4.6759) (50.3797, 4.6159) (50.2423, 4.5608) knots 0 0 0 0 1 1 1 1
  arc A321 (50.2423, 4.5608) -> (49.9925, 4.1564) centre (50.3911, 4.1895) ccw
  arc A322 (50.0343, 3.6183) -> (49.9925, 4.1564) centre (0, 0) ccw
  arc A323 (50.0343, 3.6183) -> (50.3437, 3.2573) centre (50.4333, 3.6472) ccw
  spline S322 degree 3 poles (50.3437, 3.2573) (50.4879, 3.2242) (50.6392, 3.187) (50.7973, 3.1455) knots 0 0 0 0 1 1 1 1
  spline S323 degree 3 poles (50.7973, 3.1455) (51.4203, 2.9819) (52.1476, 2.7507) (52.9672, 2.4252) knots 0 0 0 0 1 1 1 1
  circle A324 centre (0, 0) radius 5.9
  circle A325 centre (0, 0) radius 27.5
  circle A326 centre (0, 0) radius 65.0226
  circle A327 centre (0, 0) radius 65.0226
  dimension "d4" = 11.8
  dimension "d5" = 55
  measures "d4" diameter of A324
  measures "d5" diameter of A325
extrude "Extrusion2" add sketch "Skizze1 (2)" along normal blind 10 contours A0 S0 S1 A1 A2 A3 S2 S3 A4 S4 S5 A5 A6 A7 S6 S7 A8 S8 S9 A9 A10 A11 S10 S11 A12 S12 S13 A13 A14 A15 S14 S15 A16 S16 S17 A17 A18 A19 S18 S19 A20 S20 S21 A21 A22 A23 S22 S23 A24 S24 S25 A25 A26 A27 S26 S27 A28 S28 S29 A29 A30 A31 S30 S31 A32 S32 S33 A33 A34 A35 S34 S35 A36 S36 S37 A37 A38 A39 S38 S39 A40 S40 S41 A41 A42 A43 S42 S43 A44 S44 S45 A45 A46 A47 S46 S47 A48 S48 S49 A49 A50 A51 S50 S51 A52 S52 S53 A53 A54 A55 S54 S55 A56 S56 S57 A57 A58 A59 S58 S59 A60 S60 S61 A61 A62 A63 S62 S63 A64 S64 S65 A65 A66 A67 S66 S67 A68 S68 S69 A69 A70 A71 S70 S71 A72 S72 S73 A73 A74 A75 S74 S75 A76 S76 S77 A77 A78 A79 S78 S79 A80 S80 S81 A81 A82 A83 S82 S83 A84 S84 S85 A85 A86 A87 S86 S87 A88 S88 S89 A89 A90 A91 S90 S91 A92 S92 S93 A93 A94 A95 S94 S95 A96 S96 S97 A97 A98 A99 S98 S99 A100 S100 S101 A101 A102 A103 S102 S103 A104 S104 S105 A105 A106 A107 S106 S107 A108 S108 S109 A109 A110 A111 S110 S111 A112 S112 S113 A113 A114 A115 S114 S115 A116 S116 S117 A117 A118 A119 S118 S119 A120 S120 S121 A121 A122 A123 S122 S123 A124 S124 S125 A125 A126 A127 S126 S127 A128 S128 S129 A129 A130 A131 S130 S131 A132 S132 S133 A133 A134 A135 S134 S135 A136 S136 S137 A137 A138 A139 S138 S139 A140 S140 S141 A141 A142 A143 S142 S143 A144 S144 S145 A145 A146 A147 S146 S147 A148 S148 S149 A149 A150 A151 S150 S151 A152 S152 S153 A153 A154 A155 S154 S155 A156 S156 S157 A157 A158 A159 S158 S159 A160 S160 S161 A161 A162 A163 S162 S163 A164 S164 S165 A165 A166 A167 S166 S167 A168 S168 S169 A169 A170 A171 S170 S171 A172 S172 S173 A173 A174 A175 S174 S175 A176 S176 S177 A177 A178 A179 S178 S179 A180 S180 S181 A181 A182 A183 S182 S183 A184 S184 S185 A185 A186 A187 S186 S187 A188 S188 S189 A189 A190 A191 S190 S191 A192 S192 S193 A193 A194 A195 S194 S195 A196 S196 S197 A197 A198 A199 S198 S199 A200 S200 S201 A201 A202 A203 S202 S203 A204 S204 S205 A205 A206 A207 S206 S207 A208 S208 S209 A209 A210 A211 S210 S211 A212 S212 S213 A213 A214 A215 S214 S215 A216 S216 S217 A217 A218 A219 S218 S219 A220 S220 S221 A221 A222 A223 S222 S223 A224 S224 S225 A225 A226 A227 S226 S227 A228 S228 S229 A229 A230 A231 S230 S231 A232 S232 S233 A233 A234 A235 S234 S235 A236 S236 S237 A237 A238 A239 S238 S239 A240 S240 S241 A241 A242 A243 S242 S243 A244 S244 S245 A245 A246 A247 S246 S247 A248 S248 S249 A249 A250 A251 S250 S251 A252 S252 S253 A253 A254 A255 S254 S255 A256 S256 S257 A257 A258 A259 S258 S259 A260 S260 S261 A261 A262 A263 S262 S263 A264 S264 S265 A265 A266 A267 S266 S267 A268 S268 S269 A269 A270 A271 S270 S271 A272 S272 S273 A273 A274 A275 S274 S275 A276 S276 S277 A277 A278 A279 S278 S279 A280 S280 S281 A281 A282 A283 S282 S283 A284 S284 S285 A285 A286 A287 S286 S287 A288 S288 S289 A289 A290 A291 S290 S291 A292 S292 S293 A293 A294 A295 S294 S295 A296 S296 S297 A297 A298 A299 S298 S299 A300 S300 S301 A301 A302 A303 S302 S303 A304 S304 S305 A305 A306 A307 S306 S307 A308 S308 S309 A309 A310 A311 S310 S311 A312 S312 S313 A313 A314 A315 S314 S315 A316 S316 S317 A317 A318 A319 S318 S319 A320 S320 S321 A321 A322 A323 S322 S323 | A325 | A326 A327 in component "Internal Gear (81 teeth)"
extrude "Extrusion4" add sketch "Skizze1 (2)" along normal blind 30 contours A325 in component "Internal Gear (81 teeth)"
sketch "Skizze5" plane through (0, 55, 0) normal (0, 1, 0) x (-1, 0, 0)
  circle A0 centre (0, 0) radius 5.9
  circle A1 centre (0, 0) radius 27.5
  line L0 (0, 0) -> (-27.5, 0) construction
  circle A2 centre (0, 0) radius 27.5
  line L1 (-17.5, 2.25) -> (17.5, 2.25)
  line L2 (-17.5, -2.25) -> (17.5, -2.25)
  line L3 (0, 0) -> (0, 27.5) construction
  line L4 (-17.5, 2.25) -> (-17.5, -2.25)
  line L5 (17.5, 2.25) -> (17.5, -2.25)
  dimension "d24" = 4.5
  dimension "d25" = 35
  dimension "d26" = 35
  constraint coincident A0.centre A1.centre
  constraint coincident A1 L0.end
  constraint horizontal L0
  constraint parallel L0 L1
  constraint horizontal L2
  constraint symmetric L0 L1 L2
  constraint coincident A2 L3.end
  constraint perpendicular L1 L3
  constraint perpendicular L0 L4
  constraint symmetric L3 L4 L5
  measures "d24" distance of L1 L2
  measures "d25" distance of L1.start L1.end
  measures "d26" distance of L2.start L2.end
extrude "Extrusion5" cut sketch "Skizze5" against normal blind 4 contours A0 L1 L2 L5 | A0 L1 L2 L4 in component "Internal Gear (81 teeth)"
sketch "Skizze13" plane through (0, 0, 0) normal (1, 0, 0) x (0, 1, 0)
  line L0 (35, -65.0226) -> (35, 65.0226)
  line L1 (55, -27.5) -> (55, 27.5)
  line L2 (35, -65.0226) -> (55, -27.5)
  line L3 (55, -27.5) -> (35, -27.5)
  constraint coincident L0.start L2.start
  constraint coincident L1.start L2.end
  constraint coincident L0 L3.end
  constraint perpendicular L0 L3
revolve "Drehen1" add sketch "Skizze13" angle 360 about axis through (0, 25, 0) along (0, -1, 0) in component "Internal Gear (81 teeth)"
fillet "Abrundung1" radius 3 2 edges at (-60.6224, 0, 23.5132) (60.6224, 35, -23.5132) in component "Internal Gear (81 teeth)"
sketch "Skizze14" plane through (0, 0, 0) normal (1, 0, 0) x (0, 1, 0)
  line L0 (0, -65.0226) -> (0, 65.0226)
  line L1 (55, 0) -> (55, 27.5)
  line L2 (0, 0) -> (55, 0) construction
  line L3 (51, 27.5) -> (51, -25.2431) construction
  dimension "d108" = 55
  dimension "d109" = 4
  constraint coincident L2.start origin
  constraint coincident L1.start L2.end
  constraint parallel L1 L3
  measures "d108" distance of L2.start L1.start
  measures "d109" distance of L1 L3
component "Internal Gear (81 teeth)" placed x (1, 0, 0) y (0, 1, 0) z (0, 0, 1) at (0, 0, 0)
equation "d26 = d25"
named bodies: "Zahnkranz_Aquazepp"
